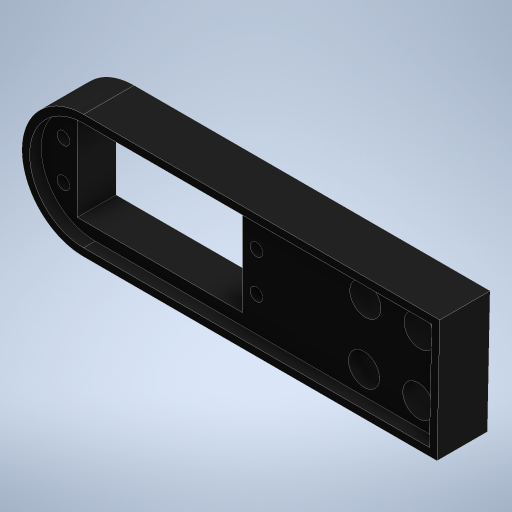
# Autodesk Inventor part: Ramie3
Saved by Autodesk Inventor 2024.2 (Build 282272000, 272)
## iProperties
Created: 2023-11-11
Part Number: Ramie3
Material: Ogólny
Document SubType Name: Modeling
Designer: nosal
Density: 1 g/cm^3
Appearance: Domyślna
Author: nosal
## iProperties of the stored document Ramie3_Drukowanie 3D.ipt
Created: 2023-11-11
Part Number: Ramie3_Drukowanie 3D
Material: Ogólny
Document SubType Name: Modeling
Designer: nosal
Density: 1 g/cm^3
Appearance: Domyślna
Author: nosal
Autodesk Inventor part; units mm, degrees
ref_plane "YZ Plane" through (0, 0, 0) normal (1, 0, 0) x (0, 1, 0)
ref_plane "XZ Plane" through (0, 0, 0) normal (0, 1, 0) x (-1, 0, 0)
ref_plane "XY Plane" through (0, 0, 0) normal (0, 0, 1) x (1, 0, 0)
sketch "Szkic1" plane through (0, 0, 0) normal (0, 0, 1) x (1, 0, 0)
  line L0 (20.3, -9.9) -> (-20.3, -9.9)
  line L1 (-20.3, -9.9) -> (-20.3, 9.9)
  line L2 (-20.3, 9.9) -> (20.3, 9.9)
  line L3 (20.3, 9.9) -> (20.3, -9.9)
  line L4 (20.3, -9.9) -> (-20.3, 9.9) construction
  line L5 (-20.3, -9.9) -> (20.3, 9.9) construction
  line L6 (21.3, 10.9) -> (-21.3, 10.9)
  line L7 (-21.3, 10.9) -> (-21.3, -10.9)
  line L8 (-21.3, -10.9) -> (21.3, -10.9)
  line L9 (21.3, -10.9) -> (21.3, 10.9)
  line L10 (0, 0) -> (24.89, 0)
  line L11 (24.89, 0) -> (24.89, 5)
  line L12 (24.89, 5) -> (24.89, -5)
  line L13 (0, 0) -> (-24.89, 0)
  line L14 (-24.89, 5) -> (-24.89, 0)
  line L15 (-24.89, 0) -> (-24.89, -5)
  circle A0 centre (-24.89, 5) radius 1.621
  circle A1 centre (-24.89, -5) radius 1.621
  circle A2 centre (24.89, -5) radius 1.621
  circle A3 centre (24.89, 5) radius 1.621
  line L16 (-26.511, 5) -> (-31.511, 5)
  line L17 (26.511, 5) -> (31.511, 5)
  line L18 (0, 10.9) -> (0, 15.9)
  line L19 (0, 15.9) -> (-16.6819, 15.9)
  line L20 (0, -10.9) -> (0, -15.9)
  line L21 (0, -15.9) -> (-16.6819, -15.9)
  line L22 (-31.511, -5.7364) -> (-31.511, 5.7364)
  line L23 (0, 15.9) -> (31.511, 15.9)
  line L24 (31.511, 15.9) -> (31.511, -15.9)
  line L25 (0, -15.9) -> (31.511, -15.9)
  circle A4 centre (-16.6819, 0) radius 15.9
  arc A5 (-32.5353, -15.867) -> (-31.511, -15.9) centre (-31.511, 0) ccw
  line L26 (31.511, -15.9) -> (74.4699, -15.9)
  line L27 (74.4699, -15.9) -> (75.153, 15.9)
  line L28 (75.153, 15.9) -> (31.511, 15.9)
  point P0 (15.7555, -15.9)
  point P1 (29.1703, -29.1056)
  dimension "d10" = 3.242
  dimension "d13" = 3.242
  dimension "d0" = 40.6
  dimension "d1" = 19.8
  dimension "d2" = 1
  dimension "d3" = 42.6
  dimension "d4" = 24.89
  dimension "d5" = 5
  dimension "d6" = 10
  dimension "d7" = 24.89
  dimension "d8" = 5
  dimension "d9" = 5
  dimension "d11" = 3.242
  dimension "d12" = 3.242
  dimension "d14" = 5
  dimension "d15" = 5
  dimension "d16" = 5
  dimension "d17" = 5
  dimension "d18" = 6.621
  dimension "d19" = 63.022
  dimension "d20" = 10.9
  dimension "d21" = 0
  constraints: 58 end point, 8 perpendicular, 7 horizontal, 6 midpoint, 6 point on circle, 5 parallel, 5 point on line, 4 centre point, 4 coincident, 3 vertical, 2 horizontal alignment, 1 tangent, 7 other
  measures "d0" distance of L1.end L2.end
  measures "d1" distance of L0.end L1.end
  measures "d2" distance between parallel lines of L2 L6
  measures "d3" distance of L6.start L6.end
  measures "d4" distance of L10.start L10.end
  measures "d5" distance of L10.end L11.end
  measures "d6" distance of L11.end L12.end
  measures "d7" distance of L10.start L13.end
  measures "d8" distance of L14.start L13.end
  measures "d9" distance of L13.end L15.end
  measures "d11" diameter of A1
  measures "d12" diameter of A2
  measures "d14" distance of L16.start L16.end
  measures "d15" distance of L17.start L17.end
  measures "d16" distance of L18.start L18.end
  measures "d17" distance of L20.start L20.end
  measures "d18" distance between parallel lines of L11 L24
  measures "d19" distance between parallel lines of L24 L22
  measures "d20" distance between parallel lines of L17 L23
  measures "d21" distance between parallel lines of L17 L16
extrude "Wyciągnięcie proste1" add sketch "Szkic1" along normal blind 10 contours A4 L22 L16 A0 L14 L13 L7 L8 | L8 L20 L21 A4 | L10 L11 A3 L17 L24 L25 L20 L8 L9 | L9 L6 L18 L23 L24 L17 A3 L11 L10 | L13 L14 A0 L16 L22 A4 L6 L7 | A4 L22 | A4 L19 L18 L6 | L24 L28 L27 L26
sketch "Szkic16" plane through (0, 0, 10) normal (0, 0, 1) x (1, 0, 0)
  line L0 (75.153, 15.9) -> (-16.6819, 15.9) projected
  arc A0 (-16.6819, 15.9) -> (-16.6819, -15.9) centre (-16.6819, 0) ccw projected
  line L1 (-16.6819, -15.9) -> (74.4699, -15.9) projected
  line L2 (74.4699, -15.9) -> (75.153, 15.9) projected
  circle A1 centre (24.89, 5) radius 1.621 projected
  circle A2 centre (24.89, -5) radius 1.621 projected
  line L3 (21.3, 10.9) -> (21.3, -10.9) projected
  line L4 (21.3, -10.9) -> (-21.3, -10.9) projected
  line L5 (-21.3, -10.9) -> (-21.3, 10.9) projected
  line L6 (-21.3, 10.9) -> (21.3, 10.9) projected
  circle A3 centre (-24.89, -5) radius 1.621 projected
  circle A4 centre (-24.89, 5) radius 1.621 projected
  line L7 (-16.6819, 13.9) -> (73.1096, 13.9)
  line L8 (73.1096, 13.9) -> (72.5124, -13.9)
  line L9 (72.5124, -13.9) -> (-16.6819, -13.9)
  arc A5 (-16.6819, 13.9) -> (-16.6819, -13.9) centre (-16.6819, 0) ccw
  point P0 (0, 0)
  dimension "d89" = 2
  constraints: 6 end point, 2 point on circle, 1 centre point, 3 other
  measures "d89" distance between parallel lines of L0 L7
extrude "Wyciągnięcie proste9" add sketch "Szkic16" along normal blind 3 contours L2 L1 A0 L0
sketch "Szkic18" plane through (0, 0, 0) normal (0, 0, -1) x (-1, 0, 0)
  line L0 (-75.153, 15.9) -> (16.6819, 15.9) projected
  line L1 (16.6819, -15.9) -> (-74.4699, -15.9) projected
  line L2 (-74.4699, -15.9) -> (-75.153, 15.9) projected
  point P0 (0, 0)
  point P1 (-66.9793, 7.9)
  point P2 (-66.6399, -7.9)
  point P3 (-52.9793, 7.9)
  point P4 (-52.6399, -7.9)
  dimension "d94" = 8
  dimension "d95" = 8
  dimension "d105" = 8
  dimension "d106" = 8
  dimension "d107" = 14
  dimension "d108" = 14
  dimension "d109" = 8
  dimension "d110" = 8
  measures "d94" distance from line of L0 point (-66.979, 7.9)
  measures "d95" distance from line of L1 point (-66.64, -7.9)
  measures "d105" distance from line of L2 point (-66.979, 7.9)
  measures "d106" distance from line of L2 point (-66.64, -7.9)
  measures "d107" distance of point (-52.979, 7.9) point (-66.979, 7.9)
  measures "d108" distance of point (-52.64, -7.9) point (-66.64, -7.9)
  measures "d109" distance from line of L1 point (-52.64, -7.9)
  measures "d110" distance from line of L0 point (-52.979, 7.9)
hole "Otwór3" at (66.9793, 7.9, 0) at (66.6399, -7.9, 0) at (52.9793, 7.9, 0) at (52.6399, -7.9, 0) direction (0, 0, 1) diameter 3.242 end through all thread size "M4x0.7" designation "M4" class "6H" standard "GB Metric profile"
sketch "Szkic19" plane through (0, 0, 10) normal (0, 0, 1) x (1, 0, 0)
  circle A0 centre (52.9793, 7.9) radius 1.621 projected
  circle A1 centre (66.9793, 7.9) radius 1.621 projected
  circle A2 centre (52.6399, -7.9) radius 1.621 projected
  circle A3 centre (52.9793, 7.9) radius 1.621 projected
  circle A4 centre (66.6399, -7.9) radius 1.621 projected
  circle A5 centre (66.9793, 7.9) radius 1.621 projected
  arc A6 (-16.6819, 13.9) -> (-16.6819, -13.9) centre (-16.6819, 0) ccw projected
  line L0 (-16.6819, -13.9) -> (72.5124, -13.9) projected
  line L1 (72.5124, -13.9) -> (73.1096, 13.9) projected
  line L2 (73.1096, 13.9) -> (-16.6819, 13.9) projected
  circle A7 centre (24.89, 5) radius 1.621 projected
  circle A8 centre (24.89, -5) radius 1.621 projected
  line L3 (21.3, 10.9) -> (21.3, -10.9) projected
  line L4 (21.3, -10.9) -> (-21.3, -10.9) projected
  line L5 (-21.3, -10.9) -> (-21.3, 10.9) projected
  line L6 (-21.3, 10.9) -> (21.3, 10.9) projected
  circle A9 centre (-24.89, -5) radius 1.621 projected
  circle A10 centre (-24.89, 5) radius 1.621 projected
  circle A11 centre (52.9793, 7.9) radius 4
  circle A12 centre (52.6399, -7.9) radius 4
  circle A13 centre (66.6399, -7.9) radius 4
  circle A14 centre (66.9793, 7.9) radius 4
  point P0 (0, 0)
  dimension "d111" = 8
  dimension "d112" = 8
  dimension "d113" = 8
  dimension "d114" = 8
  constraints: 4 centre point, 4 coincident
  measures "d111" diameter of A11
  measures "d112" diameter of A12
  measures "d113" diameter of A13
  measures "d114" diameter of A14
extrude "Wyciągnięcie proste10" cut sketch "Szkic19" against normal blind 6 contours A2 | A11 | A12 | A13 | A14
sketch "Szkic20" plane through (0, 0, 0) normal (0, 0, -1) x (-1, 0, 0)
  circle A0 centre (-52.6399, -7.9) radius 1.621 projected
  circle A1 centre (-52.9793, 7.9) radius 1.621 projected
  circle A2 centre (-66.6399, -7.9) radius 1.621 projected
  circle A3 centre (-66.9793, 7.9) radius 1.621 projected
  line L0 (-75.153, 15.9) -> (16.6819, 15.9) projected
  line L1 (-74.4699, -15.9) -> (-75.153, 15.9) projected
  line L2 (16.6819, -15.9) -> (-74.4699, -15.9) projected
  arc A4 (16.6819, -15.9) -> (16.6819, 15.9) centre (16.6819, 0) ccw projected
  circle A5 centre (-24.89, 5) radius 1.621 projected
  circle A6 centre (-24.89, -5) radius 1.621 projected
  line L3 (-21.3, 10.9) -> (-21.3, -10.9) projected
  line L4 (21.3, 10.9) -> (-21.3, 10.9) projected
  line L5 (21.3, -10.9) -> (21.3, 10.9) projected
  line L6 (-21.3, -10.9) -> (21.3, -10.9) projected
  circle A7 centre (24.89, -5) radius 1.621 projected
  circle A8 centre (24.89, 5) radius 1.621 projected
  circle A9 centre (24.89, -5) radius 3.5
  circle A10 centre (24.89, 5) radius 3.5
  circle A11 centre (-24.89, -5) radius 3.5
  circle A12 centre (-24.89, 5) radius 3.5
  point P0 (0, 0)
  dimension "d117" = 7
  dimension "d118" = 7
  dimension "d119" = 7
  dimension "d120" = 7
  constraints: 4 centre point, 4 coincident
  measures "d117" diameter of A9
  measures "d118" diameter of A10
  measures "d119" diameter of A11
  measures "d120" diameter of A12
extrude "Wyciągnięcie proste11" cut sketch "Szkic20" against normal blind 6 contours A5 | A6 | A7 | A8 | A9 | A10 | A11 | A12
equation "\"d13\" = d10"
equation "\"d11\" = d10"
equation "\"d12\" = d10"
